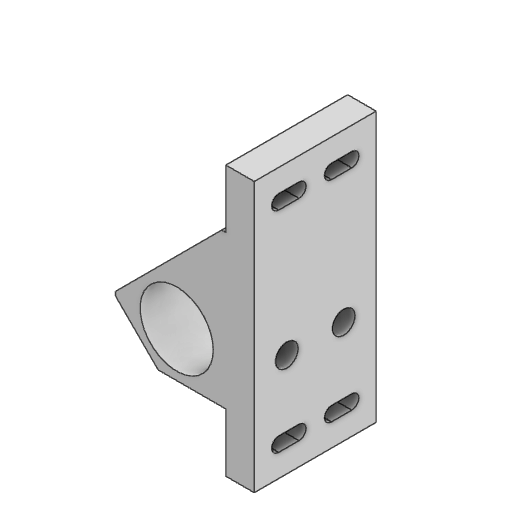
# Autodesk Inventor part: Cuvette Holder Adjustable Recv
Saved by Autodesk Inventor 2025.1 (Build 291241020, 241B)
## iProperties
Created: 2024-09-23
Part Number: Cuvette Holder Adjustable Recv
Material: Generic
Document SubType Name: Modeling
Designer: wayneslade
Density: 1 g/cm^3
Appearance: Default
Author: wayneslade
Autodesk Inventor part; units mm, degrees
ref_plane "Work Plane1" through (0, 0, 0) normal (0, 0, 1) x (1, 0, 0)
sketch "Sketch1" plane through (0, 0, 0) normal (0, 0, 1) x (1, 0, 0)
  circle A0 centre (1.7782, -8.2782) radius 7.5245 construction
  line L0 (-2.7782, -19.2782) -> (-13.7782, -8.2782) construction
  line L1 (13.7782, -19.2782) -> (-2.7782, -19.2782) construction
  line L2 (13.7782, 19.2782) -> (13.7782, -19.2782) construction
  line L3 (-13.7782, -8.2782) -> (13.7782, 19.2782) construction
  line L4 (13.8782, -19.2782) -> (-2.7782, -19.2782)
  line L5 (-2.7782, -19.2782) -> (-13.2782, -8.7782)
  circle A1 centre (1.7782, -8.2782) radius 7.5245
  line L6 (-13.2782, -7.7782) -> (12.8782, 18.3782)
  line L7 (-13.7782, -8.2782) -> (13.7782, 19.2782) construction
  line L8 (13.7782, 19.2782) -> (13.7782, 36.7218) construction
  line L9 (13.7782, 36.7218) -> (-18.2218, 36.7218) construction
  line L10 (-13.2782, -7.7782) -> (-13.2782, -8.7782)
  line L11 (20.8782, 32.7218) -> (13.8782, 32.7218)
  line L12 (13.8782, -33.6218) -> (20.8782, -33.6218)
  line L13 (20.8782, -33.6218) -> (20.8782, 32.7218)
  line L14 (13.8782, 18.3782) -> (12.8782, 18.3782)
  line L15 (13.8782, 32.7218) -> (13.8782, 18.3782)
  line L16 (13.8782, -19.2782) -> (13.8782, -33.6218)
  line L17 (13.7782, -19.2782) -> (-2.7782, -19.2782) projected
  line L18 (-2.7782, -19.2782) -> (-13.7782, -8.2782) projected
  line L19 (-18.2218, 36.7218) -> (-18.2218, -48.2782) projected
  line L20 (-18.2218, -48.2782) -> (13.7782, -48.2782) projected
  line L21 (13.7782, -48.2782) -> (13.7782, -19.2782) projected
  point P0 (0, 0)
  dimension "d0" = 0
  dimension "d4" = 0.1
  dimension "d5" = 1
  dimension "d6" = 1
  dimension "d7" = 0
  dimension "d8" = 0
  dimension "d9" = 0
  dimension "d10" = 7
  dimension "d11" = 4
  dimension "d13" = 66.3436
  constraints: 20 end point, 4 collinear, 4 parallel, 3 perpendicular, 1 centre point, 1 coincident, 1 horizontal
  measures "d0" radial gap between concentric circles of A0 A1
  measures "d4" distance between parallel lines of L8 L15
  measures "d5" distance of L14.start L6.end
  measures "d6" distance of L6.start L5.end
  measures "d7" distance between parallel lines of L3 L6
  measures "d8" distance between parallel lines of L0 L5
  measures "d9" distance between parallel lines of L1 L4
  measures "d10" distance of L11.start L11.end
  measures "d11" distance between parallel lines of L9 L11
  measures "d13" distance of L12.end L11.start
ref_plane "Work Plane2" through (-18.2218, -48.2782, 35.3062) normal (0, 0, 1) x (1, 0, 0)
extrude "Main Part Body" add sketch "Sketch1" along normal blind 35
ref_plane "Work Plane3" through (0, 0, 5) normal (0, 0, -1) x (-1, 0, 0)
sketch "Sketch2" plane through (-2.7782, -19.2782, 35) normal (0, 0, 1) x (1, 0, 0)
  circle A0 centre (4.5563, 11) radius 9
  circle A1 centre (4.5563, 11) radius 7.5245 construction
  dimension "d59" = 18
  constraints: 1 centre point, 1 coincident
  measures "d59" diameter of A0
extrude "Bore for SM05" cut sketch "Sketch2" against normal up to surface (30 mm away)
sketch "Sketch3" plane through (20.8782, -33.6218, 35.3062) normal (1, 0, 0) x (0, 0, -1)
  circle A0 centre (22.3062, 25.3437) radius 2.3
  circle A1 centre (8.3062, 25.3437) radius 2.3
  line L0 (42.3062, 25.3437) -> (-6.6938, 25.3437) construction
  line L1 (30.3062, 79.6124) -> (30.3062, -13.2687) construction
  line L2 (35.3062, 0) -> (35.3062, 66.3437) construction
  line L3 (35.3062, 66.3437) -> (0.3062, 66.3437) construction
  line L4 (0.3062, 0) -> (0.3062, 66.3437) construction
  line L5 (35.3062, 0) -> (0.3062, 0) construction
  point P0 (35.3062, 33.6218)
  dimension "d21" = 4.6
  dimension "d22" = 4.6
  dimension "d27" = 8
  dimension "d52" = 8
  constraints: 2 centre point, 2 point on line
  measures "d21" diameter of A0
  measures "d22" diameter of A1
  measures "d27" distance from line of A0.centre L1
  measures "d52" distance from line of L4 A1.centre
extrude "Thru Holes for Lens Tube Set Screws M4" cut sketch "Sketch3" against normal up to next
sketch "Sketch4" plane through (20.8782, -33.6218, 0) normal (1, 0, 0) x (0, 0, -1)
  circle A0 centre (-13, 25.3437) radius 2.3 construction
  circle A1 centre (-27, 25.3437) radius 2.3 construction
  point P0 (0, 33.6218)
hole "Holes for Set Screw Insert M4" at (20.8782, -8.2782, 13) at (20.8782, -8.2782, 27) direction (-1, 0, 0) diameter 5.6 depth 9.1
sketch "Sketch6" plane through (0, 0, 0) normal (0, 0, -1) x (-1, 0, 0)
  line L0 (-20.8782, -33.6218) -> (-20.8782, 32.7218) construction
  line L1 (-13.8782, -33.6218) -> (-20.8782, -33.6218) construction
  line L2 (-13.8782, -19.2782) -> (-13.8782, -33.6218) construction
  line L3 (2.7782, -19.2782) -> (-13.8782, -19.2782) construction
  line L4 (13.2782, -8.7782) -> (2.7782, -19.2782) construction
  line L5 (13.2782, -7.7782) -> (13.2782, -8.7782) construction
  line L6 (-12.8782, 18.3782) -> (13.2782, -7.7782) construction
  line L7 (-13.8782, 18.3782) -> (-12.8782, 18.3782) construction
  line L8 (-13.8782, 32.7218) -> (-13.8782, 18.3782) construction
  line L9 (-20.8782, 32.7218) -> (-13.8782, 32.7218) construction
  circle A0 centre (-1.7782, -8.2782) radius 7.5245 construction
  line L10 (-20.8782, 32.7218) -> (-13.8782, 32.7218)
  line L11 (-13.8782, 32.7218) -> (-13.8782, -33.6218)
  line L12 (-13.8782, -33.6218) -> (-20.8782, -33.6218)
  line L13 (-20.8782, -33.6218) -> (-20.8782, 32.7218)
  point P0 (0, 0)
  constraints: 8 end point, 2 parallel, 1 horizontal, 1 perpendicular
extrude "Extrusion5" cut sketch "Sketch6" against normal blind 5
sketch "Sketch5" plane through (20.8782, -33.6218, 0) normal (1, 0, 0) x (0, 0, -1)
  circle A0 centre (-27, 25.3437) radius 2.8 construction
  circle A1 centre (-13, 25.3437) radius 2.8 construction
  line L0 (-5, 0) -> (-35, 0) construction
  line L1 (-5, 66.3437) -> (-35, 66.3437) construction
  line L2 (0, 52) -> (-5, 52) construction
  line L3 (0, 14.3437) -> (-5, 14.3437) construction
  line L4 (0, 33.1718) -> (-35, 33.1718) construction
  line L5 (-35.6124, 59) -> (-5, 59) construction
  line L6 (-11, 59) -> (-16, 59) construction
  line L7 (-11, 60.75) -> (-16, 60.75)
  line L8 (-16, 57.25) -> (-11, 57.25)
  arc A2 (-11, 57.25) -> (-11, 60.75) centre (-11, 59) ccw
  arc A3 (-16, 60.75) -> (-16, 57.25) centre (-16, 59) ccw
  line L9 (-24, 59) -> (-29, 59) construction
  line L10 (-24, 60.75) -> (-29, 60.75)
  line L11 (-29, 57.25) -> (-24, 57.25)
  arc A4 (-24, 57.25) -> (-24, 60.75) centre (-24, 59) ccw
  arc A5 (-29, 60.75) -> (-29, 57.25) centre (-29, 59) ccw
  line L12 (-11, 5.5937) -> (-16, 5.5937)
  line L13 (-16, 9.0937) -> (-11, 9.0937)
  arc A6 (-11, 5.5937) -> (-11, 9.0937) centre (-11, 7.3437) ccw
  arc A7 (-16, 9.0937) -> (-16, 5.5937) centre (-16, 7.3437) ccw
  line L14 (-24, 5.5937) -> (-29, 5.5937)
  line L15 (-29, 9.0937) -> (-24, 9.0937)
  arc A8 (-24, 5.5937) -> (-24, 9.0937) centre (-24, 7.3437) ccw
  arc A9 (-29, 9.0937) -> (-29, 5.5937) centre (-29, 7.3437) ccw
  line L16 (-5, 0) -> (-5, 66.3437) projected
  line L17 (-35, 0) -> (-35, 66.3437) projected
  point P0 (0, 33.6218)
  point P1 (-13.5, 59)
  point P2 (-26.5, 59)
  dimension "d37" = 7
  dimension "d40" = 5
  dimension "d41" = 5
  dimension "d42" = 3.5
  dimension "d43" = 3.5
  dimension "d51" = 8
  dimension "d54" = 6
  dimension "d55" = 6
  constraints: 28 end point, 16 point on circle, 12 symmetric about line, 8 centre point, 8 tangent, 5 point on line, 3 midpoint, 3 parallel, 4 other
  measures "d37" distance between parallel lines of L2 L5
  measures "d40" distance of L6.end L6.start
  measures "d41" distance of L9.start L9.end
  measures "d42" distance between parallel lines of L8 L7
  measures "d43" distance between parallel lines of L11 L10
  measures "d51" distance of L9.start L6.end
  measures "d54" distance from line of L6.start L16
  measures "d55" distance from line of L17 L9.end
extrude "Slots for Holddown Screws" cut sketch "Sketch5" against normal through all
equation "\"d22\" = d21"
equation "\"d52\" = d27"
equation "\"d41\" = d40"
equation "\"d43\" = d42"
body "Solid1"
